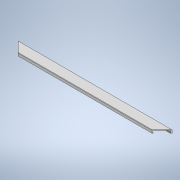
# Autodesk Inventor part: Tapa 30x30 438mm
Saved by Autodesk Inventor 2021 (Build 250183000, 183)
## iProperties
Created: 2021-04-16
Part Number: Tapa 30x30 438mm
Material: Generic
Document SubType Name: Modeling
Designer: Nelson
Density: 1 g/cm^3
Appearance: Default
Author: Nelson
Autodesk Inventor part; units mm, degrees
ref_plane "YZ Plane" through (0, 0, 0) normal (1, 0, 0) x (0, 1, 0)
ref_plane "XZ Plane" through (0, 0, 0) normal (0, 1, 0) x (-1, 0, 0)
ref_plane "XY Plane" through (0, 0, 0) normal (0, 0, 1) x (1, 0, 0)
sketch "Boceto principal" plane through (0, 0, 0) normal (1, 0, 0) x (0, 1, 0)
  line L0 (0, -1) -> (0, -3)
  line L1 (0, -3) -> (2, -3)
  line L2 (2, -3) -> (2, -2)
  line L3 (2, -2) -> (6, -2)
  line L4 (7, -3) -> (7, -27)
  line L5 (6, -28) -> (2, -28)
  line L6 (2, -28) -> (2, -27)
  line L7 (2, -27) -> (0, -27)
  line L8 (0, -27) -> (0, -29)
  line L9 (1, -30) -> (8, -30)
  line L10 (9, -29) -> (9, -1)
  line L11 (8, 0) -> (1, 0)
  arc A0 (1, 0) -> (0, -1) centre (1, -1) ccw
  arc A1 (7, -3) -> (6, -2) centre (6, -3) ccw
  arc A2 (6, -28) -> (7, -27) centre (6, -27) ccw
  arc A3 (0, -29) -> (1, -30) centre (1, -29) ccw
  arc A4 (8, -30) -> (9, -29) centre (8, -29) ccw
  arc A5 (9, -1) -> (8, 0) centre (8, -1) ccw
  constraints: 24 end point, 12 point on circle, 6 centre point
extrude "Extrusion1" add sketch "Boceto principal" along normal blind 438
sketch "Boceto esquinas" plane through (0, 0, 0) normal (0, 1, 0) x (-1, 0, 0)
  line L0 (0, 0) -> (-30, 0)
  line L1 (-30, 0) -> (0, -30)
  line L2 (0, -30) -> (0, 0)
  line L3 (-408, 0) -> (-438, 0)
  line L4 (-438, 0) -> (-438, -30)
  line L5 (-438, -30) -> (-408, 0)
  constraints: 12 end point
extrude "Extrusion2" cut sketch "Boceto esquinas" along normal blind 10
body "Solid1"
